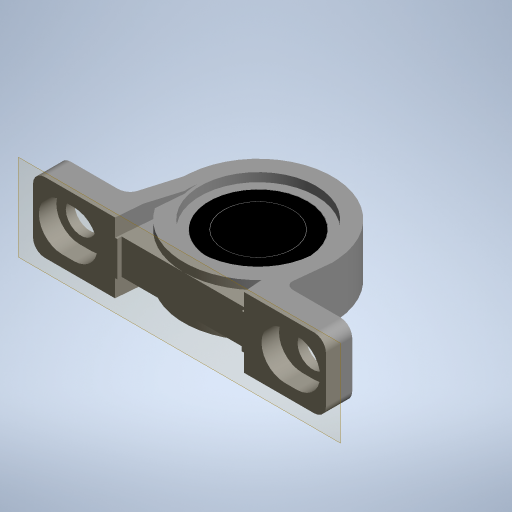
# Autodesk Inventor part: PBT10x
Saved by Autodesk Inventor 2023 (Build 270158000, 158)
## iProperties
Part Number: PBT10x
Material: 一般
Catalog Web Link: www.cadenas.de
Description: PBT, PBR, PBRS, PBRSX x-Ball Bearing Units - Pillow Type
Vendor: MISUMI
Document SubType Name: Modeling
Designer: partserver
Manufacturer: MISUMI
Mass: 12.6649 g
Surface Area: 66.1664 cm^2
Volume: 12.6649 cm^3
Density: 1 g/cm^3
Appearance: PSOLRGB-175-175-175
Category: PARTsolutions
Company: MISUMI
PSOL_IDENT_0: {$CADENAS_DATA\23d-libs\misumi\metric\12_bearing_holders\pbt.prj},175 {VTYP=3D},{NB=PBT10x},{LINA=PB
PSOL_IDENT_1: T10x},{NN=PBT, PBR, PBRS, PBRSX x},{DATE=18.06.2021 04:56:45},{GEOMDATE=08.06.2021 05:57:30},{VERSIO
PSOL_IDENT_2: N=},{LINEID=10},{WBVAR=TS,MAT},{WBNUMERIC=}  {NB=PBT10x},{LINA=PBT10x},{KT=DUMMY},{PN=PBT10},{TYPE=P
PSOL_IDENT_3: BT},{TS=T},{MAT=},{MATH=Zinc Alloy Die Cast},{MATB=52100 Bearing Steel},{MATRS=Nitrile Rubber (NBR)}
PSOL_IDENT_4: ,{MATSS=4137 Alloy Steel},{MATER=-},{STER=-},{PRECISION=JIS B 1558/JIS B 1559},{OT=-10 ~+ 80},{D=10}
PSOL_IDENT_5: ,{H=18},{L=67},{L1=53},{A=16},{DD=7},{TT=6},{TX1=6},{TX2=5},{H1=35.0},{H11=35},{H12=34.0},{B=14.0},{
PSOL_IDENT_6: B1=17.500},{B2=14.000},{S=4.0},{MASS=70},{CR=4600},{CR1=4600},{CR2=3900},{COR=2000},{COR1=2000},{COR
PSOL_IDENT_7: 2=1550},{W1=70},{W2=77},{W3=79},{D1=17.000},{D2=12.000},{D3=34.000},{D4=36.000},{D5=26.500},{M1=M3 x
PSOL_IDENT_8: 0.35},{M2=M4 x 0.7},{TT1=0.59},{TT2=1.5},{ALC1=0.35},{ALC2=0.88},{MMIN1=2.621},{MMIN2=3.242},{MMAX1=
PSOL_IDENT_9: 3.000},{MMAX2=4.000},{M=M3 x 0.35},{T=0.59},{ALC=0.35},{MMIN=2.621},{MMAX=3},{MATALG=    '','Steel'
PSOL_IDENT_10: },{X=1},{DSCREW=3},{LSCREW=4},{DS1=3.000},{LS1=4.000},{DS2=4.000},{LS2=4.000},{D6=3.500}
NB: PBT10x
NN: PBT, PBR, PBRS, PBRSX x
NT: Ball Bearing Units - Pillow Type
NBSYN: $PN.x
LINA: PBT10x
CATALOG: Misumi
TYPE: PBT
TS: Set Screw
MAT: Steel
MATH: Zinc Alloy Die Cast
MATB: 52100 Bearing Steel
MATRS: Nitrile Rubber (NBR)
MATSS: 4137 Alloy Steel
MATER: -
STER: -
PRECISION: JIS B 1558/JIS B 1559
OT: -10 ~+ 80
D: 10
H: 18
L: 67
L1: 53
A: 16
DD: 7
TT: 6
H1: 35
H11: 35
H12: 34
B: 14
S: 4
MASS: 70
CR: 4600
COR: 2000
M: M3 x 0.35
T: 0.59
ALC: 0.35
SUPPLIER: MISUMI
ARTICLENO: PBT10x
BOMINFO: PBT10x
CREATOR: CADENAS GmbH
Title: PBT10x
Author: Cadenas PARTsolutions
Comments: Ball Bearing Units - Pillow Type
Autodesk Inventor part; units mm, degrees
sketch "Sketch_1" plane through (0, 0, 0) normal (0, 0, 1) x (1, 0, 0)
  line L0 (-33.5, 6) -> (-33.5, 0)
  line L1 (-33.5, 0) -> (-14.25, 0)
  line L2 (-14.25, 0) -> (-14.25, 1)
  line L3 (-14.25, 1) -> (14.25, 1)
  line L4 (14.25, 1) -> (14.25, 0)
  line L5 (14.25, 0) -> (33.5, 0)
  line L6 (33.5, 0) -> (33.5, 6)
  line L7 (33.5, 6) -> (20.07941, 6)
  arc A0 (17.836386, 8.072964) -> (20.07941, 6) centre (20.07941, 8.25) ccw
  line L8 (17.836386, 8.072964) -> (16.947295, 19.337609)
  line L9 (16.947295, 19.337609) -> (13.848049, 19.337609)
  arc A1 (-13.848049, 19.337609) -> (13.848049, 19.337609) centre (0, 18) ccw
  line L10 (-13.848049, 19.337609) -> (-16.947295, 19.337609)
  line L11 (-16.947295, 19.337609) -> (-17.836386, 8.072964)
  arc A2 (-20.07941, 6) -> (-17.836386, 8.072964) centre (-20.07941, 8.25) ccw
  line L12 (-20.07941, 6) -> (-33.5, 6)
  constraints: 26 end point, 6 point on circle, 3 centre point
extrude "Extrusion1" add sketch "Sketch_1" along normal mid plane 16
sketch "Sketch_2" plane through (0, 0, 6) normal (0, 0, 1) x (1, 0, 0)
  line L0 (-14.737002, 0) -> (14.737002, 0)
  line L1 (14.737002, 0) -> (13.237002, 18)
  line L2 (13.237002, 18) -> (-13.237002, 18)
  line L3 (-13.237002, 18) -> (-14.737002, 0)
  constraints: 8 end point
extrude "Extrusion2" cut sketch "Sketch_2" along normal blind 8
sketch "Sketch_6" plane through (0, 0, -6) normal (0, 0, 1) x (1, 0, 0)
  line L0 (-14.737002, 0) -> (14.737002, 0)
  line L1 (14.737002, 0) -> (13.237002, 18)
  line L2 (13.237002, 18) -> (-13.237002, 18)
  line L3 (-13.237002, 18) -> (-14.737002, 0)
  constraints: 8 end point
extrude "Extrusion3" cut sketch "Sketch_6" against normal blind 8
sketch "Sketch_3" plane through (0, 0, 0) normal (1, 0, 0) x (0, 1, 0)
  line L0 (54, 32) -> (-18, 32)
  line L1 (-18, 32) -> (-18, -32)
  line L2 (-18, -32) -> (54, -32)
  line L3 (54, -32) -> (54, 32)
  line L4 (6, 8) -> (0, 8)
  line L5 (0, 8) -> (0, -8)
  line L6 (0, -8) -> (6, -8)
  line L7 (6, -8) -> (18, -6)
  line L8 (18, -6) -> (35, -6)
  line L9 (35, -6) -> (35, 6)
  line L10 (35, 6) -> (18, 6)
  line L11 (18, 6) -> (6, 8)
  constraints: 24 end point
extrude "Extrusion4" cut sketch "Sketch_3" along normal mid plane 67
sketch "Sketch_4" plane through (0, 0, 0) normal (0, 1, 0) x (-1, 0, 0)
  line L0 (134, -32) -> (134, 32)
  line L1 (134, 32) -> (-134, 32)
  line L2 (-134, 32) -> (-134, -32)
  line L3 (-134, -32) -> (134, -32)
  arc A0 (33.5, 5.32) -> (30.82, 8) centre (30.82, 5.32) ccw
  line L4 (30.82, 8) -> (-30.82, 8)
  arc A1 (-30.82, 8) -> (-33.5, 5.32) centre (-30.82, 5.32) ccw
  line L5 (-33.5, 5.32) -> (-33.5, -5.32)
  arc A2 (-33.5, -5.32) -> (-30.82, -8) centre (-30.82, -5.32) ccw
  line L6 (-30.82, -8) -> (30.82, -8)
  arc A3 (30.82, -8) -> (33.5, -5.32) centre (30.82, -5.32) ccw
  line L7 (33.5, -5.32) -> (33.5, 5.32)
  constraints: 16 end point, 8 point on circle, 4 centre point
extrude "Extrusion5" cut sketch "Sketch_4" along normal blind 6
sketch "Sketch_5" plane through (0, 0, 0) normal (1, 0, 0) x (0, 1, 0)
  line L0 (18, -4) -> (18, 10)
  line L1 (23, 10) -> (23, -4)
  line L2 (23, -4) -> (25.783333, -4)
  arc A0 (25.883333, -4) -> (25.783333, -4) centre (25.833333, -4) ccw
  line L3 (25.883333, -4) -> (29.2125, -4)
  arc A1 (29.3125, -4) -> (29.2125, -4) centre (29.2625, -4) ccw
  line L4 (29.3125, -4) -> (31.25, -4)
  line L5 (31.25, -4) -> (31.25, -6)
  line L6 (31.25, -6) -> (35, -6)
  line L7 (35, -6) -> (35, 6)
  line L8 (35, 6) -> (31.25, 6)
  line L9 (31.25, 6) -> (31.25, 4)
  line L10 (31.25, 4) -> (29.3125, 4)
  arc A2 (29.2125, 4) -> (29.3125, 4) centre (29.2625, 4) ccw
  line L11 (29.2125, 4) -> (27.166667, 4)
  line L12 (27.166667, 4) -> (27.166667, 3.333333)
  line L13 (27.166667, 3.333333) -> (25.833333, 3.333333)
  line L14 (25.833333, 3.333333) -> (25.833333, 4)
  line L15 (25.833333, 4) -> (26.5, 4)
  line L16 (26.5, 4) -> (26.5, 10)
  line L17 (26.5, 10) -> (23, 10)
  constraints: 36 end point, 6 point on circle, 3 centre point
revolve "Revolution1" add sketch "Sketch_5" angle 360 about axis through (0, 18, -4) along (0, 0, -1)
sketch "Sketch_7" plane through (0, 0, 4) normal (0, 0, 1) x (1, 0, 0)
  line L0 (-15.153668, -5) -> (15.153668, -5)
  line L1 (15.153668, -5) -> (14.036238, 8.409169)
  arc A0 (-14.036238, 8.409169) -> (14.036238, 8.409169) centre (0, 18) ccw
  line L2 (-14.036238, 8.409169) -> (-15.153668, -5)
  constraints: 6 end point, 2 point on circle, 1 centre point
extrude "Extrusion6" cut sketch "Sketch_7" along normal blind 8
sketch "Sketch_8" plane through (0, 0, -4) normal (0, 0, 1) x (1, 0, 0)
  line L0 (-15.153668, -5) -> (15.153668, -5)
  line L1 (15.153668, -5) -> (14.036238, 8.409169)
  arc A0 (-14.036238, 8.409169) -> (14.036238, 8.409169) centre (0, 18) ccw
  line L2 (-14.036238, 8.409169) -> (-15.153668, -5)
  constraints: 6 end point, 2 point on circle, 1 centre point
extrude "Extrusion7" cut sketch "Sketch_8" against normal blind 8
sketch "Sketch9" plane through (-30.82, 0, 8) normal (0, -1, 0) x (1, 0, 0)
  point P0 (4.32, -8)
hole "Hole1" at (-26.5, 0, 0) direction (0, 1, 0) diameter 7 depth 8
sketch "Sketch10" plane through (14.737002, 0, -8) normal (0, -1, 0) x (1, 0, 0)
  point P0 (11.762998, 8)
hole "Hole2" at (26.5, 0, 0) direction (0, 1, 0) diameter 7 depth 8
sketch "Sketch_13" plane through (0, 0, 0) normal (1, 0, 0) x (0, 1, 0)
  line L0 (22.5, 7.625) -> (26.5, 7.625)
  line L1 (26.5, 7.625) -> (26.5, 6.125)
  line L2 (26.5, 6.125) -> (26.2295, 6.3955)
  line L3 (26.2295, 6.3955) -> (22.7705, 6.3955)
  line L4 (22.7705, 6.3955) -> (22.5, 6.125)
  line L5 (22.5, 6.125) -> (22.5, 7.625)
  line L6 (22.5, 7.625) -> (26.5, 7.625)
  constraints: 14 end point
revolve "Revolution2" cut sketch "Sketch_13" angle 360 about axis through (0, 22.5, 7.625) along (0, -1, 0)
thread "Thread1" size "M3x0.5" class "6H" standard "ISO Metric profile" length 3.459
sketch "Sketch_11" plane through (0, 0, 0) normal (0, 1, 0) x (-1, 0, 0)
  arc A0 (32.16, 0) -> (26.826667, 5.333333) centre (26.826667, 0) ccw
  line L0 (26.826667, 5.333333) -> (24.093333, 5.333333)
  arc A1 (24.093333, 5.333333) -> (18.76, 0) centre (24.093333, 0) ccw
  arc A2 (18.76, 0) -> (24.093333, -5.333333) centre (24.093333, 0) ccw
  line L1 (24.093333, -5.333333) -> (26.826667, -5.333333)
  arc A3 (26.826667, -5.333333) -> (32.16, 0) centre (26.826667, 0) ccw
  constraints: 8 point on circle, 4 centre point, 4 end point
sketch "Sketch_12" plane through (0, 0, 0) normal (0, 1, 0) x (-1, 0, 0)
  arc A0 (-18.76, 0) -> (-24.093333, 5.333333) centre (-24.093333, 0) ccw
  line L0 (-24.093333, 5.333333) -> (-26.826667, 5.333333)
  arc A1 (-26.826667, 5.333333) -> (-32.16, 0) centre (-26.826667, 0) ccw
  arc A2 (-32.16, 0) -> (-26.826667, -5.333333) centre (-26.826667, 0) ccw
  line L1 (-26.826667, -5.333333) -> (-24.093333, -5.333333)
  arc A3 (-24.093333, -5.333333) -> (-18.76, 0) centre (-24.093333, 0) ccw
  constraints: 8 point on circle, 4 centre point, 4 end point
extrude "Extrusion8" cut sketch "Sketch_11" along normal blind 4
extrude "Extrusion9" cut sketch "Sketch_12" along normal blind 4
sketch "Sketch_21" plane through (-4.330127, 15.5, 0) normal (0.5, -0.8660254, 0) x (-0.8660254, -0.5, 0)
  line L0 (3.5, -7.625) -> (-0.5, -7.625)
  line L1 (-0.5, -7.625) -> (-0.5, -6.125)
  line L2 (-0.5, -6.125) -> (-0.2295, -6.3955)
  line L3 (-0.2295, -6.3955) -> (3.2295, -6.3955)
  line L4 (3.2295, -6.3955) -> (3.5, -6.125)
  line L5 (3.5, -6.125) -> (3.5, -7.625)
  line L6 (3.5, -7.625) -> (-0.5, -7.625)
  constraints: 14 end point
revolve "Revolution3" cut sketch "Sketch_21" angle 360 about axis through (-7.361216, 13.75, 7.625) along (-0.8660254, -0.5, 0)
thread "Thread2" size "M3x0.5" class "6H" standard "ISO Metric profile" length 3.459
ref_plane "to_screw_XY" through (0, 23, 7.625) normal (0, 1, 0) x (1, 0, 0)
ref_plane "to_screw_YZ" through (0, 23, 7.625) normal (1, 0, 0) x (0, 0, -1)
ref_plane "to_screw_ZX" through (0, 23, 7.625) normal (0, 0, -1) x (0, 1, 0)
ref_plane "to_screw_s_XY" through (-4.330127, 15.5, 7.625) normal (-0.8660254, -0.5, 0) x (0.5, -0.8660254, 0)
ref_plane "to_screw_s_YZ" through (-4.330127, 15.5, 7.625) normal (0.5, -0.8660254, 0) x (0, 0, 1)
ref_plane "to_screw_s_ZX" through (-4.330127, 15.5, 7.625) normal (0, 0, 1) x (-0.8660254, -0.5, 0)
ref_plane "作業平面7" through (33.5, 0, 5.32) normal (0, -1, 0) x (1, 0, 0)
body "Solid1"
